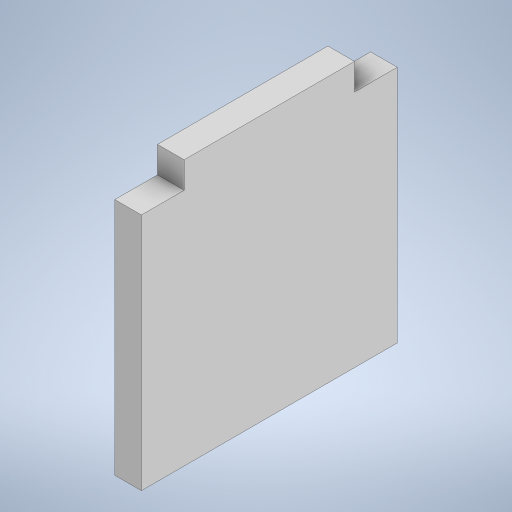
# Autodesk Inventor part: bate2
Saved by Autodesk Inventor 2024 (Build 280153000, 153)
## iProperties
Created: 2024-05-04
Part Number: bate2
Material: Generic
Document SubType Name: Modeling
Designer: samue
Density: 1 g/cm^3
Appearance: Default
Author: samue
## iProperties of the stored document bate2_3DPrint.ipt
Created: 2024-05-19
Part Number: bate2_3DPrint
Material: Generic
Document SubType Name: Modeling
Designer: samue
Density: 1 g/cm^3
Appearance: Default
Author: samue
Autodesk Inventor part; units mm, degrees
ref_plane "YZ Plane" through (0, 0, 0) normal (1, 0, 0) x (0, 1, 0)
ref_plane "XZ Plane" through (0, 0, 0) normal (0, 1, 0) x (-1, 0, 0)
ref_plane "XY Plane" through (0, 0, 0) normal (0, 0, 1) x (1, 0, 0)
sketch "Sketch1" plane through (0, 0, 0) normal (0, 1, 0) x (-1, 0, 0)
  line L0 (1.5625, 15) -> (-1.5625, 15)
  line L1 (-1.5625, 15) -> (-1.5625, -15)
  line L2 (-1.5625, -15) -> (1.5625, -15)
  line L3 (1.5625, -15) -> (1.5625, 15)
  line L4 (1.5625, 15) -> (-1.5625, -15) construction
  line L5 (-1.5625, 15) -> (1.5625, -15) construction
  point P0 (0, 0)
  dimension "d0" = 3.125
  dimension "d1" = 30
  constraints: 12 end point, 2 midpoint, 2 parallel, 1 horizontal, 1 perpendicular
  measures "d0" distance of L2.end L1.end
  measures "d1" distance of L1.end L0.end
extrude "Extrusion1" add sketch "Sketch1" along normal blind 17
sketch "Sketch3" plane through (0, 17, 0) normal (0, 1, 0) x (1, 0, 0)
  line L0 (-1.5625, -9.99) -> (1.5625, -9.99)
  line L1 (1.5625, -9.99) -> (1.5625, 9.99)
  line L2 (1.5625, 9.99) -> (-1.5625, 9.99)
  line L3 (-1.5625, 9.99) -> (-1.5625, -9.99)
  line L4 (-1.5625, -9.99) -> (1.5625, 9.99) construction
  line L5 (1.5625, -9.99) -> (-1.5625, 9.99) construction
  point P0 (0, 0)
  dimension "d4" = 3.125
  dimension "d5" = 19.98
  constraints: 12 end point, 2 midpoint, 2 parallel, 1 horizontal, 1 perpendicular
  measures "d4" distance of L2.end L1.end
  measures "d5" distance of L1.end L0.end
extrude "Extrusion2" add sketch "Sketch3" along normal blind 3.1
sketch "Sketch4" plane through (0, 0, 0) normal (0, -1, 0) x (1, 0, 0)
  line L0 (-1.5625, 15) -> (1.5625, 15) projected
  line L1 (-1.5625, -15) -> (-1.5625, -9.99) projected
  line L2 (1.5625, 15) -> (-1.5625, 15)
  line L3 (-1.5625, 15) -> (-1.5625, -15)
  line L4 (-1.5625, -15) -> (1.5625, -15)
  line L5 (1.5625, -15) -> (1.5625, 15)
  point P0 (0, 0)
  constraints: 8 end point, 2 parallel, 1 horizontal, 1 perpendicular
extrude "Extrusion3" add sketch "Sketch4" along normal blind 11
body "Solid1"
